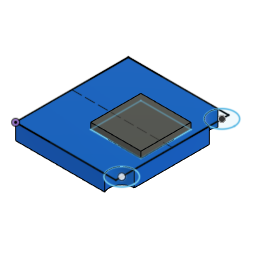
module_si7021 (Autodesk Fusion 360 design; units mm, degrees)
Autodesk Fusion 360 part; units mm, degrees
sketch "Esquisse1" plane through (0, 0, 0) normal (0, 0, 1) x (1, 0, 0)
  line L0 (0, 0) -> (8, 0)
  line L1 (8, 0) -> (8, 9)
  line L2 (8, 9) -> (0, 9)
  line L3 (0, 9) -> (0, 0)
  circle A0 centre (8, 8.4726) radius 1.0004
  circle A1 centre (8, 0.4726) radius 1.0004
  line L4 (8, 4.5) -> (0, 4.5) construction
  line L5 (7.5, 6.5) -> (3.5, 6.5)
  line L6 (3.5, 6.5) -> (3.5, 2.5)
  line L7 (3.5, 2.5) -> (7.5, 2.5)
  line L8 (7.5, 2.5) -> (7.5, 6.5)
  dimension "d1" = 8
  dimension "d2" = 9
  dimension "d3" = 4
  dimension "d4" = 4
  constraint horizontal L0
  constraint vertical L1
  constraint horizontal L2
  constraint vertical L3
  constraint coincident L0.start L3.end
  constraint coincident L1 A0.centre
  constraint midpoint L1 L4.start
  constraint midpoint L3 L4.end
  constraint horizontal L5
  constraint vertical L6
  constraint horizontal L7
  constraint vertical L8
  measures "d1" distance of L0.start L0.end
  measures "d2" distance of L0.start L2.end
  measures "d3" distance of L5.start L5.end
  measures "d4" distance of L5.start L7.end
extrude "Extrusion1" add sketch "Esquisse1" against normal blind 1.27 contours L0 L1 L2 L3 A0 A1 | L5 L6 L7 L8 makes body 1
extrude "Extrusion2" add sketch "Esquisse1" along normal blind 0.5 separate body contours L5 L6 L7 L8 makes body 2
